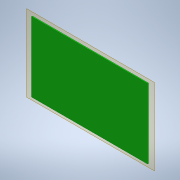
# Autodesk Inventor part: bot_layer
Saved by Autodesk Inventor 2020 (Build 240168000, 168)
## iProperties
Created: 2021-02-02
Part Number: bot_layer
Material: Generic
Document SubType Name: Modeling
Designer: phamv
Density: 1 g/cm^3
Appearance: Dark Green
Author: phamv
Autodesk Inventor part; units mm, degrees
ref_plane "YZ Plane" through (0, 0, 0) normal (1, 0, 0) x (0, 1, 0)
ref_plane "XZ Plane" through (0, 0, 0) normal (0, 1, 0) x (-1, 0, 0)
sketch "Sketch1" plane through (0, 0, 0) normal (0, 0, 1) x (1, 0, 0)
  line L0 (0, 150) -> (500, 150)
  line L1 (500, 150) -> (500, -150)
  line L2 (500, -150) -> (0, -150)
  line L3 (0, -150) -> (0, 150)
  point P0 (0, 0)
  point P1 (0, 0)
  dimension "d0" = 300
  dimension "d1" = 500
  constraints: 8 end point, 2 parallel, 1 coincident, 1 horizontal, 1 midpoint, 1 perpendicular
  measures "d0" distance between parallel lines of L2 L0
  measures "d1" distance between parallel lines of L1 L3
extrude "Extrusion1" add sketch "Sketch1" along normal blind 4
equation "\"d0\" = track_width"
equation "\"d1\" = track_length"
equation "\"d2\" = acrylic_thickness"
equation "\"track_length\" = 500"
equation "\"track_width\" = 300"
equation "\"acrylic_thickness\" = 4"
body "Solid1"
